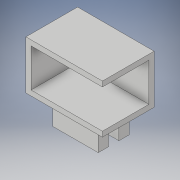
# Autodesk Inventor part: battery-holder
Saved by Autodesk Inventor 2019 (Build 230136000, 136)
## iProperties
Created: 2019-04-29
Part Number: battery-holder
Material: Generic
Document SubType Name: Modeling
Designer: Tesler
Density: 1 g/cm^3
Appearance: Default
Author: Tesler
## iProperties of the stored document battery-holder_3DPrint.ipt
Created: 2019-04-29
Part Number: battery-holder_3DPrint
Material: Generic
Document SubType Name: Modeling
Designer: Tesler
Density: 1 g/cm^3
Appearance: Default
Author: Tesler
Autodesk Inventor part; units mm, degrees
ref_plane "YZ Plane" through (0, 0, 0) normal (1, 0, 0) x (0, 1, 0)
ref_plane "XZ Plane" through (0, 0, 0) normal (0, 1, 0) x (-1, 0, 0)
ref_plane "XY Plane" through (0, 0, 0) normal (0, 0, 1) x (1, 0, 0)
sketch "Sketch1" plane through (0, 0, 0) normal (1, 0, 0) x (0, 1, 0)
  line L0 (0, 0) -> (12.5, 0)
  line L1 (12.5, 0) -> (12.5, -5)
  line L2 (12.5, -5) -> (0, -5)
  line L3 (0, 0) -> (0, 5)
  line L4 (0, 5) -> (15, 5)
  line L5 (15, 5) -> (15, -10)
  line L6 (15, -10) -> (0, -10)
  line L7 (0, -10) -> (0, -5)
  dimension "d0" = 12.5
  dimension "d2" = 5
  dimension "d3" = 15
  dimension "d4" = 15
  dimension "d5" = 5
  constraints: 16 end point, 5 perpendicular, 1 horizontal, 1 parallel, 1 point on line, 1 vertical
  measures "d0" distance of L1.end L2.end
  measures "d2" distance of L0.start L3.end
  measures "d3" distance of L3.end L4.end
  measures "d4" distance of L4.end L5.end
  measures "d5" distance of L0.end L1.end
extrude "Extrusion1" add sketch "Sketch1" along normal blind 27.5
sketch "Sketch2" plane through (0, 0, 5) normal (0, 0, 1) x (1, 0, 0)
  line L0 (0, 15) -> (27.5, 15) projected
  line L1 (0, 15) -> (0, 36)
  line L2 (0, 36) -> (2.5, 36)
  line L3 (0, 15) -> (39.5, 15)
  line L4 (39.5, 15) -> (39.5, 36)
  line L5 (39.5, 36) -> (37, 36)
  line L6 (37, 36) -> (37, 17.5)
  line L7 (37, 17.5) -> (2.5, 17.5)
  line L8 (2.5, 17.5) -> (2.5, 36)
  line L9 (0, 0) -> (27.5, 0) projected
  dimension "d8" = 21
  dimension "d9" = 2.5
  dimension "d10" = 39.5
  dimension "d11" = 2.5
  dimension "d12" = 18.5
  dimension "d13" = 17.5
  constraints: 16 end point, 4 perpendicular, 2 horizontal, 2 vertical
  measures "d8" distance of L0.start L1.end
  measures "d9" distance of L1.end L2.end
  measures "d10" distance of L0.start L3.end
  measures "d11" distance of L4.end L5.end
  measures "d12" distance of L5.end L6.end
  measures "d13" distance between parallel lines of L9 L7
extrude "Extrusion2" add sketch "Sketch2" against normal up to surface (15 mm away)
sketch "Sketch3" plane through (27.5, 0, -10) normal (0, 0, -1) x (-1, 0, 0)
  line L0 (27.5, 0) -> (22, 0)
  line L1 (22, 0) -> (22, 15)
  line L2 (22, 15) -> (27.5, 15)
  line L3 (27.5, 15) -> (27.5, 0)
  dimension "d16" = 5.5
  dimension "d17" = 15
  constraints: 8 end point, 2 parallel, 1 horizontal, 1 perpendicular
  measures "d16" distance between parallel lines of L3 L1
  measures "d17" distance between parallel lines of L2 L0
extrude "Extrusion3" cut sketch "Sketch3" against normal up to surface (15 mm away)
sketch "Sketch4" plane through (37, 17.5, -10) normal (0, 0, -1) x (-1, 0, 0)
  line L0 (-2.5, -2.5) -> (9.5, -2.5) projected
  line L1 (37, 18.5) -> (34.5, 18.5) projected
  line L2 (-2.5, -2.5) -> (37, -2.5)
  line L3 (37, -2.5) -> (37, 18.5)
  line L4 (37, 18.5) -> (-2.5, 18.5)
  line L5 (-2.5, 18.5) -> (-2.5, -2.5)
  point P0 (37, -17.5)
  constraints: 8 end point, 2 parallel, 1 horizontal, 1 perpendicular
extrude "Extrusion4" add sketch "Sketch4" along normal blind 2.5
sketch "Sketch5" plane through (2.5, 17.5, 5) normal (0, 0, 1) x (1, 0, 0)
  line L0 (37, -2.5) -> (25, -2.5) projected
  line L1 (37, 18.5) -> (37, -2.5) projected
  line L2 (34.5, 18.5) -> (37, 18.5) projected
  line L3 (34.5, 0) -> (34.5, 18.5) projected
  line L4 (0, 0) -> (34.5, 0) projected
  line L5 (0, 18.5) -> (0, 0) projected
  line L6 (-2.5, 18.5) -> (0, 18.5) projected
  line L7 (-2.5, -2.5) -> (-2.5, 18.5) projected
  line L8 (-2.5, -2.5) -> (3, -2.5) projected
  line L9 (37, 18.5) -> (37, -2.5) projected
  line L10 (37, -2.5) -> (25, -2.5) projected
  line L11 (37, 18.5) -> (34.5, 18.5)
  line L12 (34.5, 18.5) -> (34.5, 0)
  line L13 (34.5, -2.5) -> (37, -2.5)
  line L14 (37, -2.5) -> (37, 18.5)
  line L15 (0, 18.5) -> (0, 0) projected
  line L16 (-2.5, -2.5) -> (3, -2.5) projected
  line L17 (0, 18.5) -> (-2.5, 18.5)
  line L18 (-2.5, 18.5) -> (-2.5, -2.5)
  line L19 (-2.5, -2.5) -> (0, -2.5)
  line L20 (0, 0) -> (0, 18.5)
  line L21 (0, 0) -> (34.5, 0) projected
  line L22 (0, 0) -> (34.5, 0)
  line L23 (0, -2.5) -> (34.5, -2.5)
  line L24 (37, -2.5) -> (-2.5, -2.5) projected
  dimension "d22" = 34.5
  dimension "d23" = 34.5
  constraints: 20 end point, 4 parallel, 3 point on line, 2 collinear, 2 horizontal, 2 perpendicular
  measures "d22" distance between parallel lines of L5 L12
  measures "d23" distance of L19.end L13.start
extrude "Extrusion5" add sketch "Sketch5" along normal blind 2.5
sketch "Sketch6" plane through (2.5, 36, -10) normal (0, 1, 0) x (1, 0, 0)
  line L0 (37, -17.5) -> (37, 2.5) projected
  line L1 (-2.5, 2.5) -> (-2.5, -17.5) projected
  line L2 (37, 2.5) -> (-2.5, 2.5)
  line L3 (-2.5, 2.5) -> (-2.5, -17.5)
  line L4 (-2.5, -17.5) -> (37, -17.5)
  line L5 (37, -17.5) -> (37, 2.5)
  point P0 (-2.5, -10)
  constraints: 8 end point, 2 parallel, 1 horizontal, 1 perpendicular
extrude "Extrusion6" add sketch "Sketch6" along normal blind 2.5
sketch "Sketch7" plane through (2.5, 17.5, 7.5) normal (0, 0, 1) x (1, 0, 0)
  line L0 (34.5, 18.5) -> (34.5, 0) projected
  line L1 (34.5, 0) -> (0, 0) projected
  line L2 (0, 0) -> (0, 18.5) projected
  line L3 (0, 18.5) -> (34.5, 18.5) projected
  line L4 (37, -2.5) -> (37, 21) projected
  line L5 (-2.5, 21) -> (37, 21) projected
  line L6 (-2.5, -2.5) -> (-2.5, 21) projected
  line L7 (-2.5, -2.5) -> (37, -2.5) projected
  line L8 (-2.5, -2.5) -> (37, -2.5) projected
  line L9 (37, 21) -> (34.5, 21)
  line L10 (34.5, 21) -> (34.5, -2.5)
  line L11 (34.5, -2.5) -> (37, -2.5)
  line L12 (37, -2.5) -> (37, 21)
  point P0 (-2.5, -17.5)
  dimension "d28" = 2.5
  constraints: 8 end point, 2 parallel, 1 horizontal, 1 perpendicular, 1 point on line
  measures "d28" distance of L9.end L0.start
extrude "Extrusion7" cut sketch "Sketch7" against normal up to next contours L10 L5 L4 L7 L0
sketch "Sketch8" plane through (2.5, 17.5, 7.5) normal (0, 0, 1) x (1, 0, 0)
  line L0 (34.5, -2.5) -> (34.5, 0) projected
  line L1 (34.5, 0) -> (0, 0) projected
  line L2 (0, 0) -> (0, 18.5) projected
  line L3 (0, 18.5) -> (34.5, 18.5) projected
  line L4 (34.5, 18.5) -> (34.5, 21) projected
  line L5 (-2.5, 21) -> (34.5, 21) projected
  line L6 (-2.5, -2.5) -> (-2.5, 21) projected
  line L7 (-2.5, -2.5) -> (34.5, -2.5) projected
  line L8 (34.5, -2.5) -> (-2.5, -2.5)
  line L9 (-2.5, -2.5) -> (-2.5, 0)
  line L10 (0, 0) -> (34.5, 0)
  line L11 (34.5, 0) -> (34.5, -2.5)
  line L12 (34.5, 21) -> (-2.5, 21)
  line L13 (-2.5, 21) -> (-2.5, 18.5)
  line L14 (0, 18.5) -> (34.5, 18.5)
  line L15 (34.5, 18.5) -> (34.5, 21)
  line L16 (0, 18.5) -> (0, 0)
  line L17 (-2.5, 18.5) -> (-2.5, 0)
  dimension "d31" = 18.5
  constraints: 20 end point, 4 parallel, 4 point on line, 2 horizontal, 2 perpendicular, 1 collinear, 1 vertical
  measures "d31" distance between parallel lines of L14 L1
extrude "Extrusion8" add sketch "Sketch8" along normal blind 5
body "Solid1"
